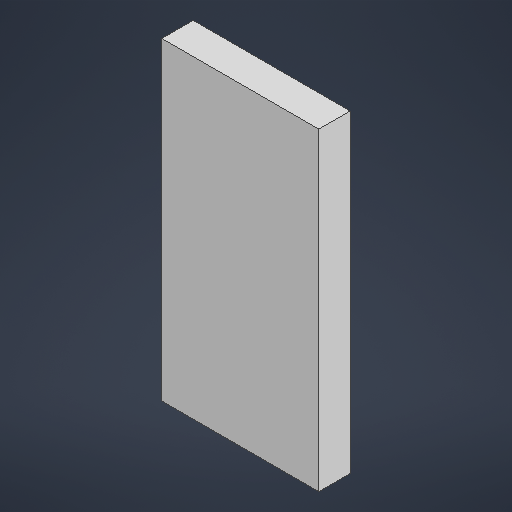
# Autodesk Inventor part: 磁铁
Saved by Autodesk Inventor 2025 (Build 290162000, 162)
## iProperties
Created: 2025-12-28
Part Number: 磁铁
Material: 常规
Document SubType Name: Modeling
Designer: XH
Density: 1 g/cm^3
Appearance: 默认
Author: XH
Autodesk Inventor part; units mm, degrees
ref_plane "YZ Plane" through (0, 0, 0) normal (1, 0, 0) x (0, 1, 0)
ref_plane "XZ Plane" through (0, 0, 0) normal (0, 1, 0) x (-1, 0, 0)
ref_plane "XY Plane" through (0, 0, 0) normal (0, 0, 1) x (1, 0, 0)
sketch "草图1" plane through (0, 0, 0) normal (0, 0, 1) x (1, 0, 0)
  line L0 (2.5, -5) -> (-2.5, -5)
  line L1 (-2.5, -5) -> (-2.5, 5)
  line L2 (-2.5, 5) -> (2.5, 5)
  line L3 (2.5, 5) -> (2.5, -5)
  line L4 (2.5, -5) -> (-2.5, 5) construction
  line L5 (-2.5, -5) -> (2.5, 5) construction
  point P0 (0, 0)
  dimension "d0" = 5
  dimension "d1" = 10
  constraints: 12 end point, 2 midpoint, 2 parallel, 1 horizontal, 1 perpendicular
  measures "d0" distance of L1.end L2.end
  measures "d1" distance of L2.end L0.start
extrude "拉伸1" add sketch "草图1" along normal blind 1
